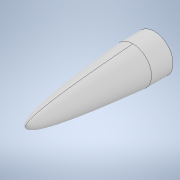
# Autodesk Inventor part: Spitze
Saved by Autodesk Inventor 2020 (Build 240168000, 168)
## iProperties
Created: 2022-01-25
Part Number: Spitze
Material: Generisch
Document SubType Name: Modeling
Designer: sp
Density: 1 g/cm^3
Appearance: Vorgabe
Author: sp
Autodesk Inventor part; units mm, degrees
ref_plane "YZ Plane" through (0, 0, 0) normal (1, 0, 0) x (0, 1, 0)
ref_plane "XZ Plane" through (0, 0, 0) normal (0, 1, 0) x (-1, 0, 0)
ref_plane "XY Plane" through (0, 0, 0) normal (0, 0, 1) x (1, 0, 0)
sketch "Skizze1" plane through (0, 0, 0) normal (1, 0, 0) x (0, 1, 0)
  line L0 (0, 2094.1927) -> (0, -1699.1575) construction
  line L1 (933.6484, 0) -> (-899.755, 0) construction
  spline S0 degree 2 poles (33, 0) (0, 400) (-33, 0) knots 0 0 0 1 1 1
  line L2 (0, 90.8614) -> (0, 0)
  line L3 (0, 0) -> (44.134, 0)
  line L4 (34.9733, 0.4054) -> (34.9733, 0)
  line L5 (-34.9733, 0.4054) -> (-34.9733, 0)
  line L6 (0, 202) -> (0, 200)
  spline S1 degree 5 poles (34.9733, 0.4054) (34.5059, 6.0674) (34.0303, 11.7288) (33.5459, 17.3894) (32.5919, 28.3221) (31.5994, 39.2514) (31.1111, 44.5218) (30.1546, 54.6264) (29.1561, 64.727) (28.6678, 69.5592) (27.7133, 78.7879) (26.7127, 88.0118) (26.2245, 92.4059) (25.2723, 100.7594) (24.2693, 109.1069) (23.7811, 113.0633) (22.8316, 120.5424) (21.8255, 128.014) (21.3374, 131.533) (20.3912, 138.1389) (19.3811, 144.7353) (18.8931, 147.8174) (17.9511, 153.5518) (16.9357, 159.2735) (16.4477, 161.9196) (15.5107, 166.7867) (14.4878, 171.6364) (13.9994, 173.849) (13.0678, 177.8573) (12.0328, 181.8401) (11.5428, 183.6233) (10.6154, 186.7902) (9.558, 189.9156) (9.0626, 191.2789) (8.1261, 193.6469) (7.016, 195.9391) (6.4972, 196.9035) (5.4731, 198.5884) (4.1868, 200.0776) (3.5562, 200.6848) (2.1324, 201.6881) (0.4393, 202.0968) (-0.4393, 202.0968) (-2.1324, 201.6881) (-3.5562, 200.6848) (-4.1868, 200.0776) (-5.4731, 198.5884) (-6.4972, 196.9035) (-7.016, 195.9391) (-8.1261, 193.6469) (-9.0626, 191.2789) (-9.558, 189.9156) (-10.6154, 186.7902) (-11.5428, 183.6233) (-12.0328, 181.8401) (-13.0678, 177.8573) (-13.9994, 173.849) (-14.4878, 171.6364) (-15.5107, 166.7867) (-16.4477, 161.9196) (-16.9357, 159.2735) (-17.9511, 153.5518) (-18.8931, 147.8174) (-19.3811, 144.7353) (-20.3912, 138.1389) (-21.3374, 131.533) (-21.8255, 128.014) (-22.8316, 120.5424) (-23.7811, 113.0633) (-24.2693, 109.1069) (-25.2723, 100.7594) (-26.2245, 92.4059) (-26.7127, 88.0118) (-27.7133, 78.7879) (-28.6678, 69.5592) (-29.1561, 64.727) (-30.1546, 54.6264) (-31.1111, 44.5218) (-31.5994, 39.2514) (-32.5919, 28.3221) (-33.5459, 17.3894) (-34.0303, 11.7288) (-34.5059, 6.0674) (-34.9733, 0.4054) knots 0 0 0 0 0 0 0.068365 0.068365 0.068365 0.132058 0.132058 0.132058 0.190501 0.190501 0.190501 0.243703 0.243703 0.243703 0.291672 0.291672 0.291672 0.334423 0.334423 0.334423 0.371973 0.371973 0.371973 0.40435 0.40435 0.40435 0.431614 0.431614 0.431614 0.453865 0.453865 0.453865 0.471312 0.471312 0.471312 0.484487 0.484487 0.484487 0.494933 0.494933 0.494933 0.505067 0.505067 0.505067 0.515513 0.515513 0.515513 0.528688 0.528688 0.528688 0.546135 0.546135 0.546135 0.568386 0.568386 0.568386 0.59565 0.59565 0.59565 0.628027 0.628027 0.628027 0.665577 0.665577 0.665577 0.708328 0.708328 0.708328 0.756297 0.756297 0.756297 0.809499 0.809499 0.809499 0.867942 0.867942 0.867942 0.931635 0.931635 0.931635 1 1 1 1 1 1
  point P0 (0, 82)
  point P1 (0, 80)
  point P2 (33, 0)
  dimension "d5" = 2
  dimension "d2" = 200
  dimension "d3" = 33
  dimension "d4" = 33
  constraints: 14 end point, 9 point on line, 3 perpendicular, 1 collinear, 1 horizontal, 1 vertical, 7 other
  measures "d2" distance of L6.end L2.end
  measures "d3" distance of L2.end point (33, 0)
  measures "d4" distance of point (-33, 0) L2.end
revolve "Umdrehung2" add sketch "Skizze1" angle 360 about axis through (0, 0, 90.8614) along (0, 0, -1)
sketch "Skizze2" plane through (0, 0, 0) normal (0, 0, -1) x (-1, 0, 0)
  circle A0 centre (0, 0) radius 33
  circle A1 centre (0, 0) radius 34.9733
  constraints: 2 centre point, 2 coincident
extrude "Extrusion1" add sketch "Skizze2" along normal blind 40
